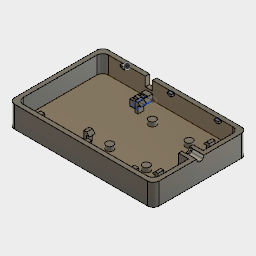
LED Light Case v8 (Autodesk Fusion 360 design; units mm, degrees)
Autodesk Fusion 360 part; units mm, degrees
sketch "Sketch1" plane through (0, 0, 0) normal (0, 1, 0) x (1, 0, 0)
  line L0 (4, 0) -> (96, 0)
  line L1 (100, 4) -> (100, 61)
  line L2 (96, 65) -> (4, 65)
  line L3 (0, 61) -> (0, 4)
  line L4 (41.61, 8.25) -> (87, 8.25)
  line L5 (87, 8.25) -> (87, 57.76)
  line L6 (87, 57.76) -> (41.61, 57.76)
  line L7 (41.61, 57.76) -> (41.61, 8.25)
  line L8 (5.6382, 56.75) -> (30.6382, 56.75)
  line L9 (30.6382, 56.75) -> (30.6382, 8.25)
  line L10 (30.6382, 8.25) -> (5.6382, 8.25)
  line L11 (5.6382, 8.25) -> (5.6382, 56.75)
  line L12 (7, 3) -> (93, 3)
  line L13 (97, 7) -> (97, 58)
  line L14 (93, 62) -> (7, 62)
  line L15 (3, 58) -> (3, 7)
  arc A0 (3, 7) -> (7, 3) centre (7, 7) ccw
  arc A1 (0, 4) -> (4, 0) centre (4, 4) ccw
  arc A2 (7, 62) -> (3, 58) centre (7, 58) ccw
  arc A3 (4, 65) -> (0, 61) centre (4, 61) ccw
  arc A4 (97, 58) -> (93, 62) centre (93, 58) ccw
  arc A5 (100, 61) -> (96, 65) centre (96, 61) ccw
  arc A6 (93, 3) -> (97, 7) centre (93, 7) ccw
  arc A7 (96, 0) -> (100, 4) centre (96, 4) ccw
  point P0 (100, 0)
  point P1 (0, 65)
  dimension "d1" = 100
  dimension "d2" = 65
  dimension "d3" = 45.39
  dimension "d4" = 49.51
  dimension "d5" = 25
  dimension "d6" = 48.5
  dimension "d11" = 5.25
  dimension "d18" = 4
  dimension "d35" = 10
  measures "d1" distance of origin P0
  measures "d2" distance of origin P1
  measures "d3" distance of L4.start L4.end
  measures "d4" distance of L4.start L6.end
  measures "d5" distance of L8.start L8.end
  measures "d6" distance of L8.start L10.end
  measures "d11" distance of L10 L12
  measures "d18" radius of A0
  measures "d35" distance of L5 L13
extrude "Extrude4" add sketch "Sketch1" along normal blind 3 contours L4 L5 L6 L7 | L8 L9 L10 L11 | L12 L13 L14 L15 A0 A2 A4 A6 makes body 1
extrude "Extrude5" add sketch "Sketch1" along normal blind 15 contours L0 L1 L2 L3 A1 A3 A5 A7 bodies 1
sketch "Sketch2" plane through (0, 3, 0) normal (0, 1, 0) x (-1, 0, 0)
  arc A0 (-93, -3) -> (-97, -7) centre (-93, -7) ccw
  line L0 (-97, -7) -> (-97, -58)
  arc A1 (-97, -58) -> (-93, -62) centre (-93, -58) ccw
  line L1 (-93, -62) -> (-7, -62)
  arc A2 (-7, -62) -> (-3, -58) centre (-7, -58) ccw
  line L2 (-3, -58) -> (-3, -7)
  arc A3 (-3, -7) -> (-7, -3) centre (-7, -7) ccw
  line L3 (-7, -3) -> (-93, -3)
  circle A4 centre (-51.61, -18.25) radius 2.5
  line L4 (-41.61, -8.25) -> (-87, -8.25)
  line L5 (-41.61, -57.76) -> (-41.61, -8.25)
  circle A5 centre (-77, -18.25) radius 2.5
  circle A6 centre (-51.61, -47.76) radius 2.5
  circle A7 centre (-77, -47.76) radius 2.5
  line L6 (-87, -8.25) -> (-87, -57.76)
  line L7 (-87, -57.76) -> (-41.61, -57.76)
  dimension "d23" = 5
  dimension "d24" = 10
  dimension "d25" = 10
  dimension "d26" = 5
  dimension "d27" = 5
  dimension "d28" = 5
  dimension "d29" = 10
  dimension "d30" = 10
  dimension "d31" = 10
  dimension "d32" = 10
  dimension "d33" = 10
  dimension "d34" = 10
  measures "d23" diameter of A4
  measures "d24" distance of A4.centre L4
  measures "d25" distance of A4.centre L5
  measures "d26" diameter of A5
  measures "d27" diameter of A6
  measures "d28" diameter of A7
  measures "d29" distance of L4 A5.centre
  measures "d30" distance of A5.centre L6
  measures "d31" distance of A6.centre L7
  measures "d32" distance of L5 A6.centre
  measures "d33" distance of A7.centre L7
  measures "d34" distance of A7.centre L6
extrude "Extrude6" add sketch "Sketch2" along normal blind 3 contours A4 | A5 | A6 | A7 bodies 1
sketch "Sketch3" plane through (0, 3, 0) normal (0, 1, 0) x (-1, 0, 0)
  circle A0 centre (-51.61, -18.25) radius 2.5
  circle A1 centre (-77, -47.76) radius 2.5
  circle A2 centre (-77, -18.25) radius 2.5
  circle A3 centre (-51.61, -47.76) radius 2.5
  arc A4 (-93, -3) -> (-97, -7) centre (-93, -7) ccw
  line L0 (-97, -7) -> (-97, -58)
  arc A5 (-97, -58) -> (-93, -62) centre (-93, -58) ccw
  line L1 (-93, -62) -> (-7, -62)
  arc A6 (-7, -62) -> (-3, -58) centre (-7, -58) ccw
  line L2 (-3, -58) -> (-3, -7)
  arc A7 (-3, -7) -> (-7, -3) centre (-7, -7) ccw
  line L3 (-7, -3) -> (-93, -3)
  line L4 (-90, -52.76) -> (-88, -52.76)
  line L5 (-88, -52.76) -> (-88, -48.76)
  line L6 (-88, -48.76) -> (-90, -48.76)
  line L7 (-90, -48.76) -> (-90, -52.76)
  line L8 (-87, -57.76) -> (-41.61, -57.76)
  line L9 (-87, -8.25) -> (-87, -57.76)
  line L10 (-88, -17.25) -> (-90, -17.25)
  line L11 (-90, -17.25) -> (-90, -13.25)
  line L12 (-90, -13.25) -> (-88, -13.25)
  line L13 (-88, -13.25) -> (-88, -17.25)
  line L14 (-41.61, -8.25) -> (-87, -8.25)
  dimension "d38" = 2
  dimension "d39" = 5
  dimension "d40" = 1
  dimension "d41" = 5
  dimension "d42" = 1
  dimension "d43" = 2
  dimension "d44" = 4
  dimension "d45" = 4
  measures "d38" distance of L4.start L4.end
  measures "d39" distance of L4 L8
  measures "d40" distance of L5 L9
  measures "d41" distance of L12 L14
  measures "d42" distance of L9 L13
  measures "d43" distance of L11.end L12.end
  measures "d44" distance of L10.end L11.end
  measures "d45" distance of L4.start L6.end
extrude "Extrude7" add sketch "Sketch3" along normal blind 7 contours L4 L5 L6 L7 | L10 L11 L12 L13 bodies 1
sketch "Sketch4" plane through (0, 10, 0) normal (0, 1, 0) x (-1, 0, 0)
  line L0 (-88, -13.25) -> (-90, -13.25)
  line L1 (-90, -13.25) -> (-90, -17.25)
  line L2 (-90, -17.25) -> (-88, -17.25)
  line L3 (-88, -17.25) -> (-88, -13.25)
  line L4 (-90, -17.25) -> (-86, -17.25)
  line L5 (-86, -17.25) -> (-86, -13.25)
  line L6 (-86, -13.25) -> (-90, -13.25)
  line L7 (-90, -13.25) -> (-90, -17.25)
  dimension "d48" = 4
  dimension "d49" = 4
  measures "d48" distance of L1.end L4.end
  measures "d49" distance of L1.end L0.end
extrude "Extrude8" add sketch "Sketch4" against normal blind 2 contours L3 L4 L5 L6 bodies 1
chamfer "Chamfer1" distance 2 angle 45 1 edges at (86, 10, -15.25) on bodies 1
sketch "Sketch5" plane through (0, 10, 0) normal (0, 1, 0) x (-1, 0, 0)
  line L0 (-90, -48.76) -> (-90, -52.76)
  line L1 (-90, -52.76) -> (-88, -52.76)
  line L2 (-88, -52.76) -> (-88, -48.76)
  line L3 (-88, -48.76) -> (-90, -48.76)
  line L4 (-90, -52.76) -> (-86, -52.76)
  line L5 (-86, -52.76) -> (-86, -48.76)
  line L6 (-86, -48.76) -> (-90, -48.76)
  line L7 (-90, -48.76) -> (-90, -52.76)
  dimension "d53" = 4
  dimension "d54" = 4
  measures "d53" distance of L0.end L4.end
  measures "d54" distance of L0.end L0.start
extrude "Extrude9" add sketch "Sketch5" against normal blind 2 contours L2 L4 L5 L6 bodies 1
chamfer "Chamfer2" distance 2 angle 45 1 edges at (86, 10, -50.76) on bodies 1
sketch "Sketch6" plane through (0, 3, 0) normal (0, 1, 0) x (-1, 0, 0)
  line L0 (-88, -13.25) -> (-88, -17.25)
  line L1 (-88, -17.25) -> (-90, -17.25)
  line L2 (-90, -17.25) -> (-90, -13.25)
  line L3 (-90, -13.25) -> (-88, -13.25)
  line L4 (-90, -48.76) -> (-88, -48.76)
  line L5 (-88, -48.76) -> (-88, -52.76)
  line L6 (-88, -52.76) -> (-90, -52.76)
  line L7 (-90, -52.76) -> (-90, -48.76)
  circle A0 centre (-51.61, -18.25) radius 2.5
  circle A1 centre (-77, -47.76) radius 2.5
  circle A2 centre (-77, -18.25) radius 2.5
  circle A3 centre (-51.61, -47.76) radius 2.5
  arc A4 (-93, -3) -> (-97, -7) centre (-93, -7) ccw
  line L8 (-97, -7) -> (-97, -58)
  arc A5 (-97, -58) -> (-93, -62) centre (-93, -58) ccw
  line L9 (-93, -62) -> (-7, -62)
  arc A6 (-7, -62) -> (-3, -58) centre (-7, -58) ccw
  line L10 (-3, -58) -> (-3, -7)
  arc A7 (-3, -7) -> (-7, -3) centre (-7, -7) ccw
  line L11 (-7, -3) -> (-93, -3)
  line L12 (-38.61, -52.76) -> (-40.61, -52.76)
  line L13 (-40.61, -52.76) -> (-40.61, -48.76)
  line L14 (-40.61, -48.76) -> (-38.61, -48.76)
  line L15 (-38.61, -48.76) -> (-38.61, -52.76)
  line L16 (-38.61, -13.25) -> (-40.61, -13.25)
  line L17 (-40.61, -13.25) -> (-40.61, -17.25)
  line L18 (-40.61, -17.25) -> (-38.61, -17.25)
  line L19 (-38.61, -17.25) -> (-38.61, -13.25)
  line L20 (-41.61, -8.25) -> (-87, -8.25)
  line L21 (-41.61, -57.76) -> (-41.61, -8.25)
  line L22 (-87, -57.76) -> (-41.61, -57.76)
  dimension "d58" = 4
  dimension "d59" = 2
  dimension "d60" = 4
  dimension "d61" = 2
  dimension "d62" = 5
  dimension "d63" = 1
  dimension "d64" = 5
  dimension "d65" = 1
  measures "d58" distance of L12.start L14.end
  measures "d59" distance of L12.start L12.end
  measures "d60" distance of L16.start L18.end
  measures "d61" distance of L16.start L16.end
  measures "d62" distance of L16 L20
  measures "d63" distance of L17 L21
  measures "d64" distance of L12 L22
  measures "d65" distance of L13 L21
extrude "Extrude10" add sketch "Sketch6" along normal blind 7 contours L12 L13 L14 L15 | L16 L17 L18 L19 bodies 1
sketch "Sketch7" plane through (0, 10, 0) normal (0, 1, 0) x (-1, 0, 0)
  line L0 (-38.61, -48.76) -> (-40.61, -48.76)
  line L1 (-40.61, -48.76) -> (-40.61, -52.76)
  line L2 (-40.61, -52.76) -> (-38.61, -52.76)
  line L3 (-38.61, -52.76) -> (-38.61, -48.76)
  line L4 (-38.61, -52.76) -> (-42.61, -52.76)
  line L5 (-42.61, -52.76) -> (-42.61, -48.76)
  line L6 (-42.61, -48.76) -> (-38.61, -48.76)
  line L7 (-38.61, -48.76) -> (-38.61, -52.76)
  dimension "d68" = 4
  dimension "d69" = 4
  measures "d68" distance of L2.end L0.start
  measures "d69" distance of L2.end L4.end
extrude "Extrude11" add sketch "Sketch7" against normal blind 2 contours L1 L4 L5 L6 bodies 1
chamfer "Chamfer3" distance 2 angle 45 1 edges at (42.61, 10, -50.76) on bodies 1
sketch "Sketch8" plane through (0, 10, 0) normal (0, 1, 0) x (-1, 0, 0)
  line L0 (-38.61, -17.25) -> (-38.61, -13.25)
  line L1 (-38.61, -13.25) -> (-40.61, -13.25)
  line L2 (-40.61, -13.25) -> (-40.61, -17.25)
  line L3 (-40.61, -17.25) -> (-38.61, -17.25)
  line L4 (-38.61, -17.25) -> (-42.61, -17.25)
  line L5 (-42.61, -17.25) -> (-42.61, -13.25)
  line L6 (-42.61, -13.25) -> (-38.61, -13.25)
  line L7 (-38.61, -13.25) -> (-38.61, -17.25)
  dimension "d73" = 4
  dimension "d74" = 4
  measures "d73" distance of L0.start L0.end
  measures "d74" distance of L0.start L4.end
extrude "Extrude12" add sketch "Sketch8" against normal blind 2 contours L2 L4 L5 L6 bodies 1
chamfer "Chamfer4" distance 2 angle 45 1 edges at (42.61, 10, -15.25) on bodies 1
sketch "Sketch12" plane through (0, 3, 0) normal (0, 1, 0) x (-1, 0, 0)
  line L0 (-38.61, -17.25) -> (-40.61, -17.25)
  line L1 (-40.61, -17.25) -> (-40.61, -13.25)
  line L2 (-40.61, -13.25) -> (-38.61, -13.25)
  line L3 (-38.61, -13.25) -> (-38.61, -17.25)
  line L4 (-38.61, -48.76) -> (-38.61, -52.76)
  line L5 (-38.61, -52.76) -> (-40.61, -52.76)
  line L6 (-40.61, -52.76) -> (-40.61, -48.76)
  line L7 (-40.61, -48.76) -> (-38.61, -48.76)
  line L8 (-88, -13.25) -> (-88, -17.25)
  line L9 (-88, -17.25) -> (-90, -17.25)
  line L10 (-90, -17.25) -> (-90, -13.25)
  line L11 (-90, -13.25) -> (-88, -13.25)
  line L12 (-90, -48.76) -> (-88, -48.76)
  line L13 (-88, -48.76) -> (-88, -52.76)
  line L14 (-88, -52.76) -> (-90, -52.76)
  line L15 (-90, -52.76) -> (-90, -48.76)
  circle A0 centre (-51.61, -18.25) radius 2.5
  circle A1 centre (-77, -47.76) radius 2.5
  circle A2 centre (-77, -18.25) radius 2.5
  circle A3 centre (-51.61, -47.76) radius 2.5
  arc A4 (-93, -3) -> (-97, -7) centre (-93, -7) ccw
  line L16 (-97, -7) -> (-97, -58)
  arc A5 (-97, -58) -> (-93, -62) centre (-93, -58) ccw
  line L17 (-93, -62) -> (-7, -62)
  arc A6 (-7, -62) -> (-3, -58) centre (-7, -58) ccw
  line L18 (-3, -58) -> (-3, -7)
  arc A7 (-3, -7) -> (-7, -3) centre (-7, -7) ccw
  line L19 (-7, -3) -> (-93, -3)
  line L20 (-97, -37.5) -> (-90, -37.5)
  line L21 (-90, -37.5) -> (-90, -27.5)
  line L22 (-90, -27.5) -> (-97, -27.5)
  line L23 (-97, -27.5) -> (-97, -37.5)
  line L24 (-93, -3) -> (-7, -3)
  point P0 (-97, -7)
  point P1 (-97, -58)
  dimension "d87" = 10
  dimension "d88" = 7
  dimension "d112" = 24.5
  measures "d87" distance of L20.start L22.end
  measures "d88" distance of L21 L23
  measures "d112" distance of L17 L20
extrude "Extrude13" add sketch "Sketch12" along normal blind 12 contours L16 L20 L21 L22 L23 bodies 1
sketch "Sketch13" plane through (90, 0, 0) normal (-1, 0, 0) x (0, 0, 1)
  line L0 (-37.5, 3) -> (-27.5, 3)
  line L1 (-27.5, 3) -> (-27.5, 15)
  line L2 (-27.5, 15) -> (-37.5, 15)
  line L3 (-37.5, 15) -> (-37.5, 3)
  circle A0 centre (-32.5, 15) radius 2.55
  dimension "d91" = 5.1
  measures "d91" diameter of A0
extrude "Extrude14" cut sketch "Sketch13" against normal blind 10 contours L2 A0 | L2 A0 bodies 1
sketch "Sketch14" plane through (90, 0, 0) normal (-1, 0, 0) x (0, 0, 1)
  arc A0 (-35.05, 15) -> (-29.95, 15) centre (-32.5, 15) ccw
  line L0 (-35.05, 15) -> (-37.5, 15)
  line L1 (-37.5, 15) -> (-37.5, 3)
  line L2 (-37.5, 3) -> (-27.5, 3)
  line L3 (-27.5, 3) -> (-27.5, 15)
  circle A1 centre (-32.5, 15) radius 2.8
  line L4 (-27.5, 15) -> (-29.95, 15)
  dimension "d95" = 5.6
  measures "d95" diameter of A1
extrude "Extrude15" cut sketch "Sketch14" against normal blind 1 from surface at -1 contours A0 L0 A1 L4 | A0 L0 A1 L4 bodies 1
sketch "Sketch15" plane through (0, 0, -62) normal (0, 0, 1) x (1, 0, 0)
  line L0 (7, 3) -> (93, 3)
  line L1 (93, 3) -> (93, 15)
  line L2 (93, 15) -> (7, 15)
  line L3 (7, 15) -> (7, 3)
  line L4 (19.9944, 15) -> (20, 15)
  line L5 (20, 15) -> (17, 15)
  line L6 (17, 15) -> (17, 14.5356)
  line L7 (18.479, 13.5) -> (20, 13.5)
  line L8 (20, 13.5) -> (20, 15)
  line L9 (17, 14.5356) -> (18.479, 13.5)
  line L10 (52.5, 13.5) -> (52.5, 15)
  line L11 (50.979, 13.5) -> (52.5, 13.5)
  line L12 (49.5, 14.5356) -> (50.979, 13.5)
  line L13 (49.5, 15) -> (49.5, 14.5356)
  line L14 (52.5, 15) -> (49.5, 15)
  line L15 (85, 13.5) -> (85, 15)
  line L16 (83.479, 13.5) -> (85, 13.5)
  line L17 (82, 14.5356) -> (83.479, 13.5)
  line L18 (82, 15) -> (82, 14.5356)
  line L19 (85, 15) -> (82, 15)
  dimension "d107" = 10
  dimension "d123" = 1.5
  dimension "d124" = 3
  dimension "d127" = 65
  dimension "d128" = 0
  dimension "d154" = 42.5
  dimension "d155" = 11
  dimension "d156" = 32.5
  measures "d107" distance of L3 L6
  measures "d123" distance of L5 L7
  measures "d124" distance of L4.end L5.end
  measures "d154" distance of L3 L13
  measures "d155" distance of L1 L18
  measures "d156" distance of L13 L18
extrude "Extrude20" add sketch "Sketch15" along normal blind 2 separate body contours L2 L4 L5 L6 L7 L8 L9 | L2 L15 L16 L17 L18 L19 | L2 L10 L11 L12 L13 L14 makes body 2 at (19, 15, -61.3333) makes body 3 at (51.5, 15, -60.6667) makes body 4 at (84, 15, -61.3333)
ref_plane "WorkPlane1" through (50, 9, -32.5) normal (0, 0, 1) x (1, 0, 0)
sketch "Sketch16" plane through (0, 3, 0) normal (0, 1, 0) x (-1, 0, 0)
  line L0 (-97, -27.5) -> (-90, -27.5)
  line L1 (-90, -27.5) -> (-90, -37.5)
  line L2 (-90, -37.5) -> (-97, -37.5)
  line L3 (-97, -37.5) -> (-97, -58)
  arc A0 (-97, -58) -> (-93, -62) centre (-93, -58) ccw
  line L4 (-93, -62) -> (-7, -62)
  arc A1 (-7, -62) -> (-3, -58) centre (-7, -58) ccw
  line L5 (-3, -58) -> (-3, -7)
  arc A2 (-3, -7) -> (-7, -3) centre (-7, -7) ccw
  line L6 (-7, -3) -> (-93, -3)
  arc A3 (-93, -3) -> (-97, -7) centre (-93, -7) ccw
  line L7 (-97, -7) -> (-97, -27.5)
  circle A4 centre (-51.61, -47.76) radius 2.5
  circle A5 centre (-77, -18.25) radius 2.5
  circle A6 centre (-77, -47.76) radius 2.5
  circle A7 centre (-51.61, -18.25) radius 2.5
  line L8 (-90, -48.76) -> (-88, -48.76)
  line L9 (-88, -48.76) -> (-88, -52.76)
  line L10 (-88, -52.76) -> (-90, -52.76)
  line L11 (-90, -52.76) -> (-90, -48.76)
  line L12 (-88, -13.25) -> (-88, -17.25)
  line L13 (-88, -17.25) -> (-90, -17.25)
  line L14 (-90, -17.25) -> (-90, -13.25)
  line L15 (-90, -13.25) -> (-88, -13.25)
  line L16 (-38.61, -48.76) -> (-38.61, -52.76)
  line L17 (-38.61, -52.76) -> (-40.61, -52.76)
  line L18 (-40.61, -52.76) -> (-40.61, -48.76)
  line L19 (-40.61, -48.76) -> (-38.61, -48.76)
  line L20 (-38.61, -17.25) -> (-40.61, -17.25)
  line L21 (-40.61, -17.25) -> (-40.61, -13.25)
  line L22 (-40.61, -13.25) -> (-38.61, -13.25)
  line L23 (-38.61, -13.25) -> (-38.61, -17.25)
  line L24 (-90, -37.5) -> (-89, -37.5)
  line L25 (-89, -37.5) -> (-89, -32.5)
  line L26 (-89, -32.5) -> (-90, -32.5)
  line L27 (-90, -32.5) -> (-90, -37.5)
  dimension "d118" = 1
  dimension "d119" = 5
  measures "d118" distance of L1.end L24.end
  measures "d119" distance of L24.end L25.end
extrude "Extrude18" add sketch "Sketch16" along normal blind 1 contours L1 L24 L25 L26 L27 bodies 1
mirror "Mirror2" about plane through (89, 3, -32.5) normal (0, 0, 1) of bodies 3 2 4 makes body 5 at (84, 15, -3.6667) makes body 6 at (19, 15, -3.6667) makes body 7 at (51.5, 15, -4.3333)
sketch "Sketch17" plane through (0, 3, 0) normal (0, 1, 0) x (-1, 0, 0)
  line L0 (-38.61, -17.25) -> (-40.61, -17.25)
  line L1 (-40.61, -17.25) -> (-40.61, -13.25)
  line L2 (-40.61, -13.25) -> (-38.61, -13.25)
  line L3 (-38.61, -13.25) -> (-38.61, -17.25)
  line L4 (-38.61, -48.76) -> (-38.61, -52.76)
  line L5 (-38.61, -52.76) -> (-40.61, -52.76)
  line L6 (-40.61, -52.76) -> (-40.61, -48.76)
  line L7 (-40.61, -48.76) -> (-38.61, -48.76)
  line L8 (-88, -13.25) -> (-88, -17.25)
  line L9 (-88, -17.25) -> (-90, -17.25)
  line L10 (-90, -17.25) -> (-90, -13.25)
  line L11 (-90, -13.25) -> (-88, -13.25)
  line L12 (-90, -48.76) -> (-88, -48.76)
  line L13 (-88, -48.76) -> (-88, -52.76)
  line L14 (-88, -52.76) -> (-90, -52.76)
  line L15 (-90, -52.76) -> (-90, -48.76)
  circle A0 centre (-51.61, -18.25) radius 2.5
  circle A1 centre (-77, -47.76) radius 2.5
  circle A2 centre (-77, -18.25) radius 2.5
  circle A3 centre (-51.61, -47.76) radius 2.5
  line L16 (-90, -32.5) -> (-89, -32.5)
  line L17 (-89, -32.5) -> (-89, -37.5)
  line L18 (-89, -37.5) -> (-97, -37.5)
  line L19 (-97, -37.5) -> (-97, -58)
  arc A4 (-97, -58) -> (-93, -62) centre (-93, -58) ccw
  line L20 (-93, -62) -> (-7, -62)
  arc A5 (-7, -62) -> (-3, -58) centre (-7, -58) ccw
  line L21 (-3, -58) -> (-3, -7)
  arc A6 (-3, -7) -> (-7, -3) centre (-7, -7) ccw
  line L22 (-7, -3) -> (-93, -3)
  arc A7 (-93, -3) -> (-97, -7) centre (-93, -7) ccw
  line L23 (-97, -7) -> (-97, -27.5)
  line L24 (-97, -27.5) -> (-90, -27.5)
  line L25 (-90, -27.5) -> (-90, -32.5)
  line L26 (-37.5361, -62) -> (-32.7361, -62)
  line L27 (-32.7361, -62) -> (-32.7361, -51)
  line L28 (-32.7361, -51) -> (-37.5361, -51)
  line L29 (-37.5361, -51) -> (-37.5361, -62)
  line L30 (-33.2361, -58.83) -> (-37.0361, -58.83)
  line L31 (-37.0361, -58.83) -> (-37.0361, -56.43)
  line L32 (-37.0361, -56.43) -> (-33.2361, -56.43)
  line L33 (-33.2361, -56.43) -> (-33.2361, -58.83)
  line L34 (-37.0361, -51) -> (-35.0361, -51)
  line L35 (-35.0361, -51) -> (-35.0361, -52.45)
  line L36 (-35.0361, -52.45) -> (-37.0361, -52.45)
  line L37 (-37.0361, -52.45) -> (-37.0361, -51)
  dimension "d134" = 4.8
  dimension "d135" = 11
  dimension "d136" = 3.8
  dimension "d137" = 3.17
  dimension "d138" = 2.4
  dimension "d145" = 0.5
  dimension "d149" = 1.45
  dimension "d150" = 2
  dimension "d151" = 0.5
  measures "d134" distance of L26.start L26.end
  measures "d135" distance of L26.start L28.end
  measures "d136" distance of L30.start L30.end
  measures "d137" distance of L26 L30
  measures "d138" distance of L30.start L32.end
  measures "d145" distance of L27 L33
  measures "d149" distance of L34.start L36.end
  measures "d150" distance of L35.end L36.end
  measures "d151" distance of L29 L37
extrude "Extrude24" add sketch "Sketch17" along normal blind 6 contours L28 L34 L35 L36 L37 bodies 1
extrude "Extrude21" add sketch "Sketch17" along normal blind 3 contours L30 L31 L32 L33 bodies 1
extrude "Extrude22" add sketch "Sketch17" along normal blind 4 contours L20 L26 L27 L28 L29 L35 L36 L37 | L28 L34 L35 L36 L37 bodies 1
sketch "Sketch18" plane through (0, 0, -62) normal (0, 0, 1) x (1, 0, 0)
  line L0 (32.5129, 15.035) -> (37.3129, 15.035)
  line L1 (37.3129, 15.035) -> (37.3129, 8.635)
  line L2 (37.3129, 8.635) -> (32.5129, 8.635)
  line L3 (32.5129, 8.635) -> (32.5129, 15.035)
  line L4 (32.7361, 7) -> (37.5361, 7)
  dimension "d143" = 6.4
  dimension "d144" = 4.8
  dimension "d146" = 1.635
  measures "d143" distance of L0.start L2.end
  measures "d144" distance of L1.end L2.end
  measures "d146" distance of L2 L4
extrude "Extrude23" cut sketch "Sketch18" against normal blind 3 bodies 1
